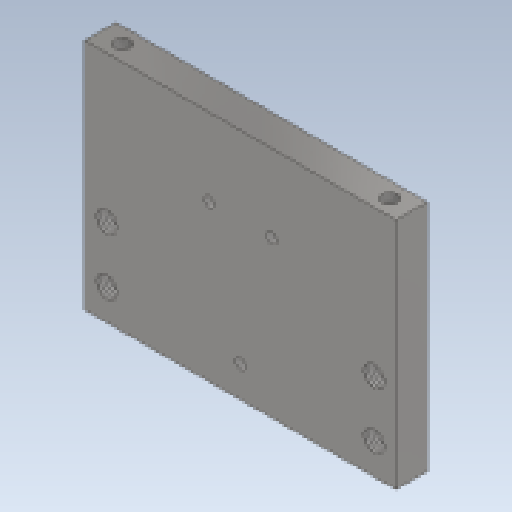
# Autodesk Inventor part: Lift_adaptor
Saved by Autodesk Inventor 2025.2 (Build 292293000, 293)
## iProperties
Created: 2025-05-09
Part Number: Lift_adaptor
Material: Stainless Steel
Document SubType Name: Modeling
Designer: Sergio Quintero
Density: 8 g/cm^3
Appearance: Semi-Polished
Author: Sergio Quintero
Autodesk Inventor part; units mm, degrees
ref_plane "YZ Plane" through (0, 0, 0) normal (1, 0, 0) x (0, 1, 0)
ref_plane "XZ Plane" through (0, 0, 0) normal (0, 1, 0) x (-1, 0, 0)
ref_plane "XY Plane" through (0, 0, 0) normal (0, 0, 1) x (1, 0, 0)
sketch "Sketch1" plane through (0, 0, 0) normal (0, 0, 1) x (1, 0, 0)
  line L0 (50, -30) -> (-50, -30)
  line L1 (-50, -30) -> (-50, 30)
  line L2 (-50, 30) -> (50, 30)
  line L3 (50, 30) -> (50, -30)
  line L4 (50, -30) -> (-50, 30) construction
  line L5 (-50, -30) -> (50, 30) construction
  line L6 (-70, 0) -> (70, 0) projected
  line L7 (-50, 30) -> (50, 30)
  line L8 (50, 30) -> (50, 45)
  line L9 (50, 45) -> (-50, 45)
  line L10 (-50, 45) -> (-50, 30)
  point P0 (0, 0)
  dimension "d2" = 100
  dimension "d3" = 60
  dimension "d45" = 15
  constraints: 20 end point, 4 parallel, 2 horizontal, 2 midpoint, 2 perpendicular, 1 other
  measures "d2" distance of L1.end L2.end
  measures "d3" distance of L0.end L1.end
  measures "d45" distance of L8.end L7.end
extrude "Extrusion1" add sketch "Sketch1" along normal blind 10 contours L0 L1 L6 L3 | L6 L1 L2 L3
sketch "Sketch2" plane through (0, 0, 10) normal (0, 0, 1) x (1, 0, 0)
  line L0 (-43, -20) -> (43, -20) construction
  line L1 (43, -20) -> (43, -2) construction
  line L2 (43, -2) -> (-43, -2) construction
  line L3 (-43, -2) -> (-43, -20) construction
  line L4 (-50, -30) -> (50, -30) construction
  line L5 (0, -42) -> (0, 42) construction
  point P0 (0, 0)
  dimension "d6" = 86
  dimension "d7" = 18
  dimension "d8" = 10
  constraints: 8 end point, 4 coincident, 2 parallel, 1 horizontal, 1 perpendicular, 1 other
  measures "d6" distance of L2.end L1.end
  measures "d7" distance of L1.end L0.end
  measures "d8" distance between parallel lines of L4 L0
hole "Hole1" at (-43, -2, 10) at (43, -2, 10) at (43, -20, 10) at (-43, -20, 10) direction (0, 0, -1) diameter 6.647 end through all thread size "M8x1.25" class "6H" standard "ISO Metric profile"
sketch "Sketch3" plane through (0, 0, 10) normal (0, 0, 1) x (1, 0, 0)
  line L0 (50, 30) -> (-50, 30) projected
  line L1 (0, -42) -> (0, 42) projected
  point P0 (0, 0)
  point P1 (-10, 20)
  point P2 (10, 20)
  point P3 (0, -20)
  dimension "d16" = 10
  dimension "d17" = 10
  dimension "d18" = 40
  constraints: 1 point on line, 1 symmetric about line
  measures "d16" distance from line of point (-10, 20) L0
  measures "d17" horizontal distance of point (0, 0) point (-10, 20)
  measures "d18" vertical distance of point (0, -20) point (10, 20)
hole "Hole4" at (-10, 20, 10) at (10, 20, 10) at (0, -20, 10) direction (0, 0, -1) diameter 3.242 end through all thread size "M4x0.7" class "6H" standard "ISO Metric profile"
extrude "Extrusion3" add sketch "Sketch1" along normal blind 10 contours L2 L10 L9 L8
sketch "Sketch5" plane through (-50, 45, 0) normal (0, 1, 0) x (1, 0, 0)
  line L0 (0, -10) -> (100, -10) construction
  line L1 (50, -10) -> (50, 0) construction
  line L2 (48.379, 0) -> (48.379, -10) construction
  point P0 (93, -5)
  point P1 (7, -5)
  dimension "d48" = 5
  dimension "d49" = 86
  constraints: 2 end point, 1 midpoint, 1 parallel, 1 symmetric about line
  measures "d48" distance from line of L0 point (93, -5)
  measures "d49" distance of point (7, -5) point (93, -5)
hole "Hole5" at (43, 45, 5) at (-43, 45, 5) direction (0, -1, 0) diameter 4.917 depth 15 tip angle 118 thread size "M6x1" class "6H" standard "ISO Metric profile"
body "Solid1"
